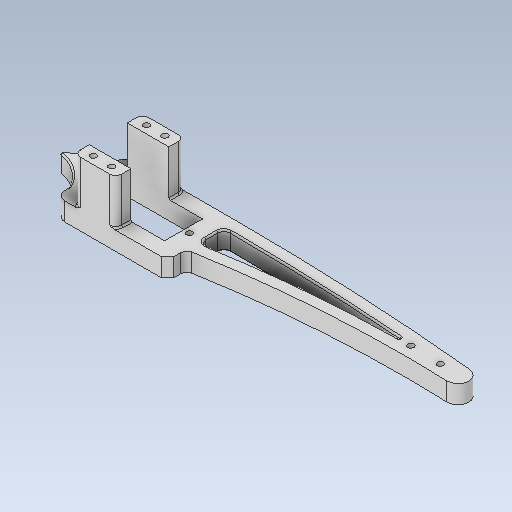
# Autodesk Inventor part: LegEnd_Right_v1
Saved by Autodesk Inventor 2020.3 (Build 243373000, 373)
## iProperties
Created: 2021-02-18
Part Number: LegEnd_Right_v1
Material: Generic
Document SubType Name: Modeling
Designer: sanyi
Density: 1 g/cm^3
Appearance: Default
Author: sanyi
Autodesk Inventor part; units mm, degrees
ref_plane "YZ Plane" through (0, 0, 0) normal (1, 0, 0) x (0, 1, 0)
ref_plane "XZ Plane" through (0, 0, 0) normal (0, 1, 0) x (-1, 0, 0)
ref_plane "XY Plane" through (0, 0, 0) normal (0, 0, 1) x (1, 0, 0)
sketch "Sketch1" plane through (0, 0, 0) normal (0, 1, 0) x (-1, 0, 0)
  line L0 (0, 0) -> (-4, 0)
  line L1 (0, 0) -> (0, 36.6)
  line L2 (-22.4, 0) -> (-22.4, 36.6)
  line L3 (-17.4, 6) -> (-5, 6)
  line L4 (-5, 6) -> (-5, 30.6)
  line L5 (-5, 30.6) -> (-17.4, 30.6)
  line L6 (-17.4, 30.6) -> (-17.4, 6)
  line L7 (-22.4, 36.6) -> (-18.4, 36.6) construction
  arc A0 (-15.1221, 113.1021) -> (-18.4834, 116.9404) centre (-15, 116.6) ccw
  arc A1 (-18.4834, 116.9404) -> (-22.4, 36.6) centre (803.5628, 36.6) ccw
  line L8 (-11.2, 4.1) -> (-11.2, 32.5) construction
  line L9 (-26.8761, 4.1) -> (8.0494, 4.1) construction
  line L10 (-27.3708, 32.5) -> (4.7796, 32.5) construction
  line L11 (-27.5308, 18.3) -> (1.4723, 18.3) construction
  arc A2 (-11.5026, 116.4641) -> (-6, 36.6) centre (360.8103, 101.9949) ccw
  arc A3 (-16.2077, 96.5934) -> (-18.4, 36.6) centre (803.5628, 36.6) ccw
  arc A4 (-15.745, 96.6) -> (-10.0624, 36.6) centre (360.8103, 101.9949) ccw
  line L12 (-18.4, 36.6) -> (-10.0624, 36.6)
  line L13 (-6, 36.6) -> (0, 36.6)
  line L14 (-16.2077, 96.5934) -> (-15.745, 96.6)
  line L15 (-15.745, 96.6) -> (-11.7455, 96.6573) construction
  line L16 (-16.2077, 96.5934) -> (-20.197, 96.8853) construction
  line L17 (-10.0624, 36.6) -> (-6.1232, 37.2946) construction
  line L18 (-15, 116.6) -> (-11.5, 116.6) construction
  line L19 (-15, 116.6) -> (-15.5584, 100.6097) construction
  line L20 (-17.4, 6) -> (-22.4, 6)
  line L21 (-5, 6) -> (0, 6)
  arc A5 (-15.4, 0) -> (-14.1296, -5.6127) centre (-2.3667, 0) ccw
  arc A6 (-9.6573, 0) -> (-14.1296, -5.6127) centre (-0.4435, -11.9298) ccw
  arc A7 (-18.4, 0) -> (-13, -12) centre (-2.3667, 0) ccw
  arc A8 (-4, 0) -> (-13, -12) centre (1.9602, -13.8452) ccw
  line L22 (-14.1296, -5.6127) -> (-16.8371, -6.9046) construction
  line L23 (-14.1296, -5.6127) -> (-11.4588, -6.9792) construction
  line L24 (-18.4, 0) -> (-22.4, 0)
  line L25 (-15.4, 0) -> (-18.4, 0) construction
  line L26 (-9.6573, 0) -> (-15.4, 0)
  line L27 (-7.7289, -2.2981) -> (-9.6573, 0) construction
  arc A9 (-18.4834, 116.9404) -> (-15.1221, 113.1021) centre (-15, 116.6) ccw
  line L28 (-19.9, -3.4679) -> (-19.9, 37.7463) construction
  line L29 (-22.4, 19.6) -> (-17.4, 19.6)
  line L30 (-5, 19.6) -> (0, 19.6)
  line L31 (-29.0378, 12.8) -> (2.5913, 12.8) construction
  point P0 (-15.2094, 110.6037)
  dimension "d4" = 6
  dimension "d5" = 24.6
  dimension "d6" = 12.4
  dimension "d7" = 5
  dimension "d15" = 7
  dimension "d17" = 6
  dimension "d18" = 4
  dimension "d21" = 20
  dimension "d23" = 80
  dimension "d24" = 15
  dimension "d29" = 170
  dimension "d30" = 6
  dimension "d31" = 10
  dimension "d43" = 4
  dimension "d44" = 3
  dimension "d45" = 4
  dimension "d50" = 13
  dimension "d51" = 12
  dimension "d52" = 130
  dimension "d53" = 92
  dimension "d89" = 6.8
  dimension "d90" = 28.4
  constraints: 64 end point, 28 point on circle, 15 point on line, 14 line through centre, 10 centre point, 9 horizontal, 6 equal length, 6 perpendicular, 4 vertical, 3 parallel, 3 tangent, 2 collinear, 1 equal radius, 8 other
  measures "d4" distance between parallel lines of L0 L3
  measures "d5" distance between parallel lines of L5 L3
  measures "d6" distance between parallel lines of L4 L6
  measures "d7" distance between parallel lines of L1 L4
  measures "d15" diameter of A0
  measures "d17" distance of L1.end L13.start
  measures "d18" distance of L2.end L7.end
  measures "d21" vertical distance of L18.start L14.end
  measures "d23" vertical distance of L18.start L1.end
  measures "d24" horizontal distance of L1.end L18.start
  measures "d29" angle of L12 L17
  measures "d30" distance of L18.start point (-15.209, 110.604)
  measures "d31" distance of L19.end point (-15.209, 110.604)
  measures "d43" distance of L2.start L24.start
  measures "d44" distance of L25.start L24.start
  measures "d45" distance of L0.start L0.end
  measures "d50" distance from line of L1 A7.end
  measures "d51" distance from line of L24 A7.end
  measures "d52" angle of L26 L27
  measures "d53" angle of L18 L19
  measures "d89" distance between parallel lines of L3 L31
  measures "d90" distance between parallel lines of L9 L10
extrude "Extrusion1" add sketch "Sketch1" along normal blind 6 contours L0 A8 A7 L24 L2 L20 L3 L21 L1 | L30 L4 L5 L6 L29 L2 A1 A9 A0 A2 L13 L1 | A0 A9
fillet "Fillet1" radius 3 1 edges at (22.4, 3, 0)
fillet "Fillet1" radius 3 1 edges at (0, 3, 0)
full round fillet "Fillet2" first side at (18.3729, 2, 43.2718) centre faces at (16.0535, 2, 96.5956) second side at (13.775, 4, 63.1507)
fillet "Fillet3" radius 2 3 edges at (18.4, 3, 36.6) (10.0624, 3, 36.6) (6, 3, 36.6)
hole "Hole1" at (11.2, 0, 4.1) at (11.2, 0, 32.5) direction (0, 1, 0) diameter 2 end through all
fillet "Fillet4" radius 0.5 1 edges at (13, 3, -12)
hole "Hole2" at (15.5584, 0, 100.6097) at (15.2094, 0, 110.6037) direction (0, 1, 0) diameter 2 end through all
extrude "Extrusion3" add sketch "Sketch1" along normal blind 20.92 contours L21 L4 L30 L1 | L20 L2 L29 L6
sketch "Sketch3" plane through (0, 20.92, 0) normal (0, 1, 0) x (1, 0, 0)
  line L0 (22.4, -19.6) -> (22.4, -6) projected
  line L1 (0, -6) -> (0, -19.6) projected
  line L2 (29.0378, -12.8) -> (-2.5913, -12.8) construction
  line L3 (19.9, -9.8) -> (19.9, -15.8) construction
  line L4 (19.9, -15.8) -> (2.5, -15.8) construction
  line L5 (2.5, -15.8) -> (2.5, -9.8) construction
  line L6 (2.5, -9.8) -> (19.9, -9.8) construction
  line L7 (11.2, -4.1) -> (11.2, -32.5) construction
  line L8 (17.4, -19.6) -> (17.4, -6) construction
  point P0 (0, 0)
  dimension "d91" = 6
  constraints: 10 end point, 2 parallel, 1 vertical, 3 other
  measures "d91" distance of L3.start L3.end
hole "Hole5" at (19.9, 20.92, 9.8) at (19.9, 20.92, 15.8) at (2.5, 20.92, 9.8) at (2.5, 20.92, 15.8) direction (0, -1, 0) diameter 2 depth 10 tip angle 118
fillet "Fillet5" radius 2 4 edges at (0, 13.46, 6) (22.4, 13.46, 6) (0, 13.46, 19.6) (22.4, 13.46, 19.6)
chamfer "Chamfer2" distance 2 angle 45 1 edges at (0, 3, 36.6)
fillet "Fillet8" radius 0.5 8 edges at (18.9, 6, 6) (21.8142, 6, 6.5858) (0.5858, 6, 6.5858) (3.5, 6, 6) (3.5, 6, 19.6) (0.5858, 6, 19.0142) (21.8142, 6, 19.0142) (18.9, 6, 19.6)
fillet "Fillet9" radius 0.5 26 edges at (17.8135, 6, 37.1875) (17.8185, 6, 67.5125) (16.1511, 6, 96.5334) (15.8118, 6, 96.5313) (14.2052, 6, 67.5507) (10.9102, 6, 37.3096) (14.4179, 6, 36.6) (17.8135, 0, 37.1875) (17.8185, 0, 67.5125) (16.1511, 0, 96.5334) (15.8118, 0, 96.5313) (14.2052, 0, 67.5507) (10.9102, 0, 37.3096) (14.4179, 0, 36.6) (12.5286, 6, 0) (12.2323, 0, -2.5363) (12.2323, 6, -2.5363) (15.0784, 6, -2.8773) (15.0784, 0, -2.8773) (12.5286, 0, 0) (13.2006, 6, -11.4632) (17.179, 6, -6.1369) (9.8128, 6, -4.4319) (13.2006, 0, -11.4632) (17.179, 0, -6.1369) (9.8128, 0, -4.4319)
body "Solid1"
